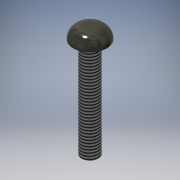
# Autodesk Inventor part: SB　18mmなべネジ
Saved by Autodesk Inventor 2020.2 (Build 242310000, 310)
## iProperties
Created: 2014-02-15
Part Number: SB　18mmなべネジ
Material: Steel, Mild
Document SubType Name: Modeling
Designer: shiota
Mass: 1.33459 g
Surface Area: 2.45934 cm^2
Volume: 0.170012 cm^3
Density: 7.85 g/cm^3
Appearance: ガンメタル
Author: shiota
Autodesk Inventor part; units mm, degrees
ref_plane "YZ Plane" through (0, 0, 0) normal (1, 0, 0) x (0, 1, 0)
ref_plane "XZ Plane" through (0, 0, 0) normal (0, 1, 0) x (-1, 0, 0)
ref_plane "XY Plane" through (0, 0, 0) normal (0, 0, 1) x (1, 0, 0)
sketch "スケッチ1" plane through (0, 0, 0) normal (0, 0, 1) x (1, 0, 0)
  circle A0 centre (0, 0) radius 1.5
  dimension "d0" = 3
  constraints: 1 centre point, 1 coincident
  measures "d0" diameter of A0
extrude "押し出し1" add sketch "スケッチ1" along normal blind 6
sketch "スケッチ2" plane through (0, 0, 6) normal (0, 0, 1) x (1, 0, 0)
  circle A0 centre (0, 0) radius 1.5 projected
  circle A1 centre (0, 0) radius 3
  dimension "d3" = 6
  constraints: 1 centre point, 1 coincident
  measures "d3" diameter of A1
extrude "押し出し2" add sketch "スケッチ2" along normal blind 2 contours A0 | A1
fillet "フィレット1" radius 2 1 edges at (-3, 0, 8)
thread "ねじ1" size "M3x0.5" class "6g" standard "ANSI Metric M Profile" full length
sketch "スケッチ3" plane through (0, 0, 0) normal (0, 0, -1) x (-1, 0, 0)
  circle A0 centre (0, 0) radius 1.5 projected
extrude "押し出し3" add sketch "スケッチ3" along normal blind 9
sketch "スケッチ4" plane through (0, 0, -9) normal (0, 0, -1) x (-1, 0, 0)
  circle A0 centre (0, 0) radius 1.5 projected
extrude "押し出し4" add sketch "スケッチ4" along normal blind 3
